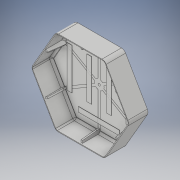
# Autodesk Inventor part: Base v5 - 175
Saved by Autodesk Inventor 2019 (Build 230136000, 136)
## iProperties
Created: 2021-07-14
Part Number: Base v5 - 175
Material: Generic
Document SubType Name: Modeling
Designer: Lix
Density: 1 g/cm^3
Appearance: Default
Author: Lix
## iProperties of the stored document Base v5 - 175_3DPrint.ipt
Created: 2021-08-05
Part Number: Base v5 - 175_3DPrint
Material: Generic
Document SubType Name: Modeling
Designer: Lix
Density: 1 g/cm^3
Appearance: Default
Author: Lix
Autodesk Inventor part; units mm, degrees
sketch "Sketch1" plane through (0, 0, 0) normal (0, 0, 1) x (1, 0, 0)
  line L0 (50.5181, -87.5) -> (-50.5181, -87.5)
  line L1 (-50.5181, -87.5) -> (-101.0363, 0)
  line L2 (-101.0363, 0) -> (-50.5181, 87.5)
  line L3 (-50.5181, 87.5) -> (50.5181, 87.5)
  line L4 (50.5181, 87.5) -> (101.0363, 0)
  line L5 (101.0363, 0) -> (50.5181, -87.5)
  point P0 (0, 0)
  point P1 (0, 0)
  point P2 (0, 0)
  dimension "d0" = 175
  constraints: 12 end point, 2 coincident, 1 horizontal, 13 other
  measures "d0" distance between parallel lines of L5 L2
extrude "Extrusion1" add sketch "Sketch1" along normal blind 40
shell "Shell1" thickness 1.5 removed faces 1 at (16.8394, -29.1667, 40) ; own thickness 1 on faces at (16.8394, -29.1667, 0)
sketch "Sketch11" plane through (-49.6521, -86, 1) normal (0, 0, 1) x (1, 0, 0)
  line L0 (-16.0979, 43.5) -> (-6.0979, 43.5)
  line L1 (-6.0979, 43.5) -> (-6.0979, 128.5)
  line L2 (-6.0979, 128.5) -> (-16.0979, 128.5)
  line L3 (-16.0979, 128.5) -> (-16.0979, 43.5)
  line L4 (-16.0979, 43.5) -> (-6.0979, 128.5) construction
  line L5 (-6.0979, 43.5) -> (-16.0979, 128.5) construction
  line L6 (24.4021, 43.5) -> (34.4021, 43.5)
  line L7 (34.4021, 43.5) -> (34.4021, 128.5)
  line L8 (34.4021, 128.5) -> (24.4021, 128.5)
  line L9 (24.4021, 43.5) -> (34.4021, 128.5) construction
  line L10 (34.4021, 43.5) -> (24.4021, 128.5) construction
  line L11 (24.4021, 128.5) -> (24.4021, 43.5)
  line L12 (64.9021, 43.5) -> (74.9021, 43.5)
  line L13 (74.9021, 43.5) -> (74.9021, 128.5)
  line L14 (74.9021, 128.5) -> (64.9021, 128.5)
  line L15 (64.9021, 43.5) -> (74.9021, 128.5) construction
  line L16 (74.9021, 43.5) -> (64.9021, 128.5) construction
  line L17 (64.9021, 128.5) -> (64.9021, 43.5)
  line L18 (105.4021, 43.5) -> (115.4021, 43.5)
  line L19 (115.4021, 43.5) -> (115.4021, 128.5)
  line L20 (115.4021, 128.5) -> (105.4021, 128.5)
  line L21 (105.4021, 43.5) -> (115.4021, 128.5) construction
  line L22 (115.4021, 43.5) -> (105.4021, 128.5) construction
  line L23 (105.4021, 128.5) -> (105.4021, 43.5)
  line L24 (-11.0979, 86) -> (110.4021, 86) construction
  line L25 (7.1521, 16) -> (92.1521, 16)
  line L26 (92.1521, 16) -> (92.1521, 26)
  line L27 (92.1521, 26) -> (7.1521, 26)
  line L28 (7.1521, 26) -> (7.1521, 16)
  line L29 (7.1521, 16) -> (92.1521, 26) construction
  line L30 (92.1521, 16) -> (7.1521, 26) construction
  line L31 (49.6521, 21) -> (49.6521, 151) construction
  line L32 (7.1521, 146) -> (92.1521, 146)
  line L33 (92.1521, 146) -> (92.1521, 156)
  line L34 (92.1521, 156) -> (7.1521, 156)
  line L35 (7.1521, 156) -> (7.1521, 146)
  line L36 (7.1521, 146) -> (92.1521, 156) construction
  line L37 (92.1521, 146) -> (7.1521, 156) construction
  point P0 (49.6521, 86)
  point P1 (29.4021, 86)
  point P2 (69.9021, 86)
  point P3 (49.6521, 86)
  dimension "d138" = 10
  dimension "d139" = 85
  dimension "d142" = 40.5
  dimension "d147" = 130
  constraints: 76 end point, 14 midpoint, 6 parallel, 5 horizontal, 4 equal length, 3 perpendicular, 1 coincident, 1 collinear, 1 horizontal alignment, 1 vertical, 32 other
  measures "d138" distance of L1.end L2.end
  measures "d139" distance of L2.end L0.start
  measures "d142" distance of L0.end L6.end
  measures "d147" distance of L31.start L31.end
extrude "Extrusion9" add sketch "Sketch11" along normal blind 0.5
ref_plane "Work Plane1" through (-25.2591, 43.75, 40) normal (0.8660254, 0.5, 0) x (0, 0, -1)
ref_plane "Work Plane2" through (-50.5181, 0, 0) normal (0, 1, 0) x (1, 0, 0)
ref_plane "Work Plane3" through (-25.2591, -43.75, 0) normal (-0.8660254, 0.5, 0) x (0, 0, 1)
sketch "Sketch12" plane through (-49.6521, -86, 1) normal (0, 0, 1) x (1, 0, 0)
  line L0 (7.1521, 16) -> (7.1521, 26) projected
  line L1 (7.1521, 26) -> (92.1521, 26) projected
  line L2 (92.1521, 26) -> (92.1521, 16) projected
  line L3 (92.1521, 16) -> (7.1521, 16) projected
  line L4 (64.9021, 43.5) -> (64.9021, 128.5) projected
  line L5 (64.9021, 128.5) -> (74.9021, 128.5) projected
  line L6 (74.9021, 128.5) -> (74.9021, 43.5) projected
  line L7 (74.9021, 43.5) -> (64.9021, 43.5) projected
  line L8 (-16.0979, 43.5) -> (-16.0979, 128.5) projected
  line L9 (-16.0979, 128.5) -> (-6.0979, 128.5) projected
  line L10 (-6.0979, 128.5) -> (-6.0979, 43.5) projected
  line L11 (-6.0979, 43.5) -> (-16.0979, 43.5) projected
  line L12 (24.4021, 43.5) -> (24.4021, 128.5) projected
  line L13 (24.4021, 128.5) -> (34.4021, 128.5) projected
  line L14 (34.4021, 128.5) -> (34.4021, 43.5) projected
  line L15 (34.4021, 43.5) -> (24.4021, 43.5) projected
  line L16 (105.4021, 43.5) -> (105.4021, 128.5) projected
  line L17 (105.4021, 128.5) -> (115.4021, 128.5) projected
  line L18 (115.4021, 128.5) -> (115.4021, 43.5) projected
  line L19 (115.4021, 43.5) -> (105.4021, 43.5) projected
  line L20 (7.1521, 146) -> (7.1521, 156) projected
  line L21 (7.1521, 156) -> (92.1521, 156) projected
  line L22 (92.1521, 156) -> (92.1521, 146) projected
  line L23 (92.1521, 146) -> (7.1521, 146) projected
  line L24 (99.3042, 0) -> (0, 0) projected
  line L25 (148.9564, 86) -> (99.3042, 0) projected
  line L26 (99.3042, 172) -> (148.9564, 86) projected
  line L27 (0, 172) -> (99.3042, 172) projected
  line L28 (-49.6521, 86) -> (0, 172) projected
  line L29 (0, 0) -> (-49.6521, 86) projected
  point P0 (49.6521, 86)
sketch "Sketch4" plane through (-49.6521, -86, 1) normal (0, 0, 1) x (1, 0, 0)
  line L0 (99.3042, 0) -> (0, 0) projected
  line L1 (148.9564, 86) -> (99.3042, 0) projected
  line L2 (99.3042, 172) -> (148.9564, 86) projected
  line L3 (0, 172) -> (99.3042, 172) projected
  line L4 (-49.6521, 86) -> (0, 172) projected
  line L5 (0, 0) -> (-49.6521, 86) projected
  line L6 (-19.2831, 128.6007) -> (2.8868, 167)
  line L7 (2.8868, 167) -> (47.2265, 167)
  line L8 (99.3042, 172) -> (0, 0) construction
  arc A0 (47.2265, 95.7014) -> (42.4633, 92.9514) centre (49.6521, 86) ccw
  line L9 (-19.2831, 128.6007) -> (42.4633, 92.9514)
  line L10 (47.2265, 167) -> (47.2265, 95.7014)
  circle A1 centre (49.6521, 86) radius 2.5
  arc A2 (40.0377, 88.75) -> (40.0377, 83.25) centre (49.6521, 86) ccw
  line L11 (-21.7088, 124.3993) -> (40.0377, 88.75)
  line L12 (-21.7088, 47.6007) -> (40.0377, 83.25)
  line L13 (-21.7088, 47.6007) -> (-43.8786, 86)
  line L14 (-43.8786, 86) -> (-21.7088, 124.3993)
  arc A3 (42.4633, 79.0486) -> (47.2265, 76.2986) centre (49.6521, 86) ccw
  line L15 (-19.2831, 43.3993) -> (42.4633, 79.0486)
  line L16 (47.2265, 5) -> (47.2265, 76.2986)
  line L17 (47.2265, 5) -> (2.8868, 5)
  line L18 (2.8868, 5) -> (-19.2831, 43.3993)
  arc A4 (52.0778, 76.2986) -> (56.8409, 79.0486) centre (49.6521, 86) ccw
  line L19 (52.0778, 5) -> (52.0778, 76.2986)
  line L20 (118.5874, 43.3993) -> (56.8409, 79.0486)
  line L21 (118.5874, 43.3993) -> (96.4175, 5)
  line L22 (96.4175, 5) -> (52.0778, 5)
  arc A5 (59.2666, 83.25) -> (59.2666, 88.75) centre (49.6521, 86) ccw
  line L23 (121.013, 47.6007) -> (59.2666, 83.25)
  line L24 (121.013, 124.3993) -> (59.2666, 88.75)
  line L25 (121.013, 124.3993) -> (143.1829, 86)
  line L26 (143.1829, 86) -> (121.013, 47.6007)
  arc A6 (56.8409, 92.9514) -> (52.0778, 95.7014) centre (49.6521, 86) ccw
  line L27 (118.5874, 128.6007) -> (56.8409, 92.9514)
  line L28 (52.0778, 167) -> (52.0778, 95.7014)
  line L29 (52.0778, 167) -> (96.4175, 167)
  line L30 (96.4175, 167) -> (118.5874, 128.6007)
  point P0 (-49.6521, 86)
  point P1 (0, 0)
  point P2 (99.3042, 0)
  point P3 (148.9564, 86)
  point P4 (99.3042, 172)
  dimension "d37" = 5
  dimension "d44" = 10
  dimension "d45" = 60
  dimension "d46" = 90
  dimension "d47" = 90
  dimension "d52" = 5.5
  dimension "d55" = 5
  dimension "d72" = 360
  constraints: 50 end point, 12 point on circle, 7 centre point, 2 equal length, 1 coincident, 1 midpoint, 73 other
  measures "d37" distance between parallel lines of L3 L7
  measures "d44" radius of A0
  measures "d45" angle of L10 L9
  measures "d46" angle of L9 L6
  measures "d47" angle of L10 L7
  measures "d52" distance of L10.end L9.end
  measures "d55" diameter of A1
extrude "Extrusion5" cut sketch "Sketch4" against normal blind 0.01 contours L6 L7 L10 A0 L9 | A1 | A2 L12 L13 L14 L11 | A3 L16 L17 L18 L15 | A4 L20 L21 L22 L19 | A5 L24 L25 L26 L23 | A6 L28 L29 L30 L27
sketch "Sketch8" plane through (-49.6521, -86, 1) normal (0, 0, 1) x (1, 0, 0)
  line L0 (99.3042, 0) -> (0, 0) projected
  line L1 (148.9564, 86) -> (99.3042, 0) projected
  line L2 (99.3042, 172) -> (148.9564, 86) projected
  line L3 (0, 172) -> (99.3042, 172) projected
  line L4 (-49.6521, 86) -> (0, 172) projected
  line L5 (0, 0) -> (-49.6521, 86) projected
  line L6 (48.1521, 164) -> (51.1521, 164)
  line L7 (51.1521, 164) -> (51.1521, 172)
  line L8 (51.1521, 172) -> (48.1521, 172)
  line L9 (48.1521, 172) -> (48.1521, 164)
  line L10 (0, 172) -> (99.3042, 172) projected
  line L11 (49.6521, 86) -> (49.6521, 172)
  point P0 (49.6521, 86)
  point P1 (49.6521, 172)
  dimension "d57" = 3
  dimension "d58" = 8
  constraints: 10 end point, 2 midpoint, 2 parallel, 1 coincident, 1 collinear, 1 horizontal, 1 perpendicular, 1 vertical
  measures "d57" distance of L6.start L6.end
  measures "d58" distance of L6.end L7.end
extrude "Extrusion6" add sketch "Sketch8" along normal blind 36 contours L7 L6 L11 L3 | L3 L11 L6 L9
sketch "Sketch9" plane through (1.5, 78, 1) normal (1, 0, 0) x (0, 0, -1)
  line L0 (0, 0) -> (0, 8) projected
  line L1 (0, 0) -> (-36, 0) projected
  line L2 (-36, 8) -> (-36, 0) projected
  line L3 (0, 8) -> (-36, 8) projected
  line L4 (-36, 8) -> (-36, 0) projected
  line L5 (-36, 0) -> (-6, 0)
  line L6 (0, 0) -> (-36, 0) projected
  line L7 (-6, 0) -> (-36, 3)
  line L8 (-36, 3) -> (-36, 0)
  point P0 (1, -78)
  point P1 (-36, 8)
  dimension "d77" = 3
  dimension "d78" = 30
  constraints: 6 end point, 3 point on line, 1 collinear, 1 perpendicular
  measures "d77" distance of L7.end L5.start
  measures "d78" distance of L5.start L5.end
extrude "Extrusion8" cut sketch "Sketch9" against normal blind 20 contours L1 L2 L7
pattern_circular "Circular Pattern1" count 6 over 360 about axis through (0, 0, 1) along (0, 0, -1) of "Extrusion6", "Extrusion8"
fillet "Fillet1" radius 4 18 edges at (-25.5761, -86, 1) (25.5761, -86, 1) (-87.2662, -20.8505, 1) (-61.6902, -65.1495, 1) (61.6902, -65.1495, 1) (87.2662, -20.8505, 1) (87.2662, 20.8505, 1) (61.6902, 65.1495, 1) (25.5761, 86, 1) (-25.5761, 86, 1) (-61.6902, 65.1495, 1) (-87.2662, 20.8505, 1) (-99.3042, 0, 20.5) (-49.6521, 86, 20.5) (49.6521, 86, 20.5) (99.3042, 0, 20.5) (49.6521, -86, 20.5) (-49.6521, -86, 20.5)
fillet "Fillet2" radius 10 6 edges at (101.0363, 0, 20) (50.5181, 87.5, 20) (-50.5181, 87.5, 20) (50.5181, -87.5, 20) (-101.0363, 0, 20) (-50.5181, -87.5, 20)
fillet "Fillet4" radius 2 5 edges at (-7.1888, 6.9514, 0.995) (-2.4257, 9.7014, 0.995) (-2.4257, 81, 0.995) (-46.7654, 81, 0.995) (-68.9352, 42.6007, 0.995)
sketch "Sketch5" plane through (-44.7446, 87.5, 0) normal (0, 1, 0) x (1, 0, 0)
  line L0 (0, 0) -> (89.4893, 0) projected
  line L1 (0, -40) -> (0, 0) projected
  point P0 (44.7446, 0)
  point P1 (44.7446, -20)
  point P2 (44.7446, 0)
  point P3 (0, -20)
  constraints: 2 midpoint, 1 horizontal alignment, 1 vertical alignment
sketch "Sketch6" plane through (53.4049, 82.5, 40) normal (0.8660254, 0.5, 0) x (0, 0, -1)
  line L0 (40, 8.6603) -> (0, 8.6603) projected
  point P0 (40, -44.7446)
  point P1 (20, -44.7446)
  point P2 (20, 8.6603)
  constraints: 1 horizontal alignment, 1 midpoint, 1 vertical alignment
sketch "Sketch7" plane through (53.4049, -82.5, 40) normal (0.8660254, -0.5, 0) x (0, 0, -1)
  line L0 (0, -8.6603) -> (40, -8.6603) projected
  point P0 (40, 44.7446)
  point P1 (20, 44.7446)
  point P2 (20, -8.6603)
  constraints: 1 horizontal alignment, 1 midpoint, 1 vertical alignment
sketch "Sketch13" plane through (0, 0, 40) normal (0, 0, 1) x (1, 0, 0)
  line L0 (-65.75, -42.5) -> (-55.75, -42.5) projected
  line L1 (-55.75, -42.5) -> (-55.75, 42.5) projected
  line L2 (-55.75, 42.5) -> (-65.75, 42.5) projected
  line L3 (-65.75, 42.5) -> (-65.75, -42.5) projected
  line L4 (-25.25, -42.5) -> (-15.25, -42.5) projected
  line L5 (-15.25, -42.5) -> (-15.25, 42.5) projected
  line L6 (-15.25, 42.5) -> (-25.25, 42.5) projected
  line L7 (-25.25, 42.5) -> (-25.25, -42.5) projected
  line L8 (-42.5, 60) -> (42.5, 60) projected
  line L9 (42.5, 60) -> (42.5, 70) projected
  line L10 (42.5, 70) -> (-42.5, 70) projected
  line L11 (-42.5, 70) -> (-42.5, 60) projected
  line L12 (15.25, -42.5) -> (25.25, -42.5) projected
  line L13 (25.25, -42.5) -> (25.25, 42.5) projected
  line L14 (25.25, 42.5) -> (15.25, 42.5) projected
  line L15 (15.25, 42.5) -> (15.25, -42.5) projected
  line L16 (55.75, -42.5) -> (65.75, -42.5) projected
  line L17 (65.75, -42.5) -> (65.75, 42.5) projected
  line L18 (65.75, 42.5) -> (55.75, 42.5) projected
  line L19 (55.75, 42.5) -> (55.75, -42.5) projected
  line L20 (-42.5, -70) -> (42.5, -70) projected
  line L21 (42.5, -70) -> (42.5, -60) projected
  line L22 (42.5, -60) -> (-42.5, -60) projected
  line L23 (-42.5, -60) -> (-42.5, -70) projected
  arc A0 (-53.4049, -82.5) -> (-44.7446, -87.5) centre (-44.7446, -77.5) ccw projected
  line L24 (-44.7446, -87.5) -> (44.7446, -87.5) projected
  arc A1 (44.7446, -87.5) -> (53.4049, -82.5) centre (44.7446, -77.5) ccw projected
  line L25 (53.4049, -82.5) -> (98.1495, -5) projected
  arc A2 (98.1495, -5) -> (98.1495, 5) centre (89.4893, 0) ccw projected
  line L26 (98.1495, 5) -> (53.4049, 82.5) projected
  arc A3 (53.4049, 82.5) -> (44.7446, 87.5) centre (44.7446, 77.5) ccw projected
  line L27 (44.7446, 87.5) -> (-44.7446, 87.5) projected
  arc A4 (-44.7446, 87.5) -> (-53.4049, 82.5) centre (-44.7446, 77.5) ccw projected
  line L28 (-53.4049, 82.5) -> (-98.1495, 5) projected
  arc A5 (-98.1495, 5) -> (-98.1495, -5) centre (-89.4893, 0) ccw projected
  line L29 (-98.1495, -5) -> (-53.4049, -82.5) projected
  line L30 (-50.8068, -84) -> (-98.1495, -2) projected
  arc A6 (-98.1495, 2) -> (-98.1495, -2) centre (-94.6854, 0) ccw projected
  line L31 (-98.1495, 2) -> (-50.8068, 84) projected
  arc A7 (-47.3427, 86) -> (-50.8068, 84) centre (-47.3427, 82) ccw projected
  line L32 (-47.3427, 86) -> (47.3427, 86) projected
  arc A8 (50.8068, 84) -> (47.3427, 86) centre (47.3427, 82) ccw projected
  line L33 (50.8068, 84) -> (98.1495, 2) projected
  arc A9 (98.1495, -2) -> (98.1495, 2) centre (94.6854, 0) ccw projected
  line L34 (98.1495, -2) -> (50.8068, -84) projected
  arc A10 (47.3427, -86) -> (50.8068, -84) centre (47.3427, -82) ccw projected
  line L35 (47.3427, -86) -> (-47.3427, -86) projected
  arc A11 (-50.8068, -84) -> (-47.3427, -86) centre (-47.3427, -82) ccw projected
  line L36 (1.5, -81) -> (-1.5, -81) projected
  line L37 (-1.5, -81) -> (-1.5, -86) projected
  line L38 (1.5, -86) -> (-1.5, -86) projected
  line L39 (1.5, -86) -> (1.5, -81) projected
  line L40 (-69.3981, -41.799) -> (-70.8981, -39.201) projected
  line L41 (-70.8981, -39.201) -> (-75.2282, -41.701) projected
  line L42 (-73.7282, -44.299) -> (-75.2282, -41.701) projected
  line L43 (-73.7282, -44.299) -> (-69.3981, -41.799) projected
  line L44 (-66.8, -40.299) -> (-69.3981, -41.799) projected
  line L45 (-68.3, -37.701) -> (-66.8, -40.299) projected
  line L46 (-70.8981, -39.201) -> (-68.3, -37.701) projected
  line L47 (-69.3981, -41.799) -> (-70.8981, -39.201) projected
  line L48 (1.5, -78) -> (1.5, -81) projected
  line L49 (-1.5, -78) -> (1.5, -78) projected
  line L50 (-1.5, -81) -> (-1.5, -78) projected
  line L51 (1.5, -81) -> (-1.5, -81) projected
  line L52 (-70.8981, 39.201) -> (-69.3981, 41.799) projected
  line L53 (-69.3981, 41.799) -> (-73.7282, 44.299) projected
  line L54 (-75.2282, 41.701) -> (-73.7282, 44.299) projected
  line L55 (-75.2282, 41.701) -> (-70.8981, 39.201) projected
  line L56 (-68.3, 37.701) -> (-70.8981, 39.201) projected
  line L57 (-66.8, 40.299) -> (-68.3, 37.701) projected
  line L58 (-69.3981, 41.799) -> (-66.8, 40.299) projected
  line L59 (-70.8981, 39.201) -> (-69.3981, 41.799) projected
  line L60 (-1.5, 81) -> (1.5, 81) projected
  line L61 (1.5, 81) -> (1.5, 86) projected
  line L62 (-1.5, 86) -> (1.5, 86) projected
  line L63 (-1.5, 86) -> (-1.5, 81) projected
  line L64 (-1.5, 78) -> (-1.5, 81) projected
  line L65 (1.5, 78) -> (-1.5, 78) projected
  line L66 (1.5, 81) -> (1.5, 78) projected
  line L67 (-1.5, 81) -> (1.5, 81) projected
  line L68 (69.3981, 41.799) -> (70.8981, 39.201) projected
  line L69 (70.8981, 39.201) -> (75.2282, 41.701) projected
  line L70 (73.7282, 44.299) -> (75.2282, 41.701) projected
  line L71 (73.7282, 44.299) -> (69.3981, 41.799) projected
  line L72 (66.8, 40.299) -> (69.3981, 41.799) projected
  line L73 (68.3, 37.701) -> (66.8, 40.299) projected
  line L74 (70.8981, 39.201) -> (68.3, 37.701) projected
  line L75 (69.3981, 41.799) -> (70.8981, 39.201) projected
  line L76 (70.8981, -39.201) -> (69.3981, -41.799) projected
  line L77 (69.3981, -41.799) -> (73.7282, -44.299) projected
  line L78 (75.2282, -41.701) -> (73.7282, -44.299) projected
  line L79 (75.2282, -41.701) -> (70.8981, -39.201) projected
  line L80 (68.3, -37.701) -> (70.8981, -39.201) projected
  line L81 (66.8, -40.299) -> (68.3, -37.701) projected
  line L82 (69.3981, -41.799) -> (66.8, -40.299) projected
  line L83 (70.8981, -39.201) -> (69.3981, -41.799) projected
  point P0 (0, 0)
body "Solid1"
